Autodesk Fusion 360 part; units mm, degrees
(part 2 of 2)
  spline S185 degree 3 poles (48.0194, -47.8906) (48.2316, -47.8906) (48.3986, -47.7898) (48.5208, -47.5882) knots 0 0 0 0 1 1 1 1
  spline S186 degree 3 poles (48.5208, -47.5882) (48.6431, -47.3867) (48.704, -47.1092) (48.704, -46.7557) knots 0 0 0 0 1 1 1 1
  spline S187 degree 3 poles (48.704, -46.7557) (48.704, -46.4046) (48.6431, -46.1283) (48.5208, -45.9268) knots 0 0 0 0 1 1 1 1
  spline S188 degree 3 poles (48.5208, -45.9268) (48.3986, -45.7252) (48.2316, -45.6244) (48.0194, -45.6244) knots 0 0 0 0 1 1 1 1
  line L174 (46.6928, -45.3714) -> (46.6928, -45.6523)
  line L175 (46.6928, -45.6523) -> (45.7067, -46.5528)
  spline S189 degree 3 poles (45.7067, -46.5528) (45.5889, -46.6608) (45.493, -46.7557) (45.4192, -46.8375) knots 0 0 0 0 1 1 1 1
  spline S190 degree 3 poles (45.4192, -46.8375) (45.3454, -46.9194) (45.2911, -46.9995) (45.2564, -47.0775) knots 0 0 0 0 1 1 1 1
  spline S191 degree 3 poles (45.2564, -47.0775) (45.2216, -47.1557) (45.2043, -47.2419) (45.2043, -47.3362) knots 0 0 0 0 1 1 1 1
  spline S192 degree 3 poles (45.2043, -47.3362) (45.2043, -47.5074) (45.2548, -47.6426) (45.356, -47.7418) knots 0 0 0 0 1 1 1 1
  spline S193 degree 3 poles (45.356, -47.7418) (45.457, -47.841) (45.5957, -47.8906) (45.7718, -47.8906) knots 0 0 0 0 1 1 1 1
  spline S194 degree 3 poles (45.7718, -47.8906) (45.9616, -47.8906) (46.1085, -47.8327) (46.2128, -47.7167) knots 0 0 0 0 1 1 1 1
  spline S195 degree 3 poles (46.2128, -47.7167) (46.317, -47.6007) (46.369, -47.4441) (46.369, -47.2469) knots 0 0 0 0 1 1 1 1
  line L176 (46.369, -47.2469) -> (46.6816, -47.2469)
  spline S196 degree 3 poles (46.6816, -47.2469) (46.6816, -47.4317) (46.6441, -47.5948) (46.5691, -47.7362) knots 0 0 0 0 1 1 1 1
  spline S197 degree 3 poles (46.5691, -47.7362) (46.494, -47.8777) (46.3883, -47.9883) (46.2518, -48.0683) knots 0 0 0 0 1 1 1 1
  spline S198 degree 3 poles (46.2518, -48.0683) (46.1154, -48.1484) (45.956, -48.1883) (45.7737, -48.1883) knots 0 0 0 0 1 1 1 1
  spline S199 degree 3 poles (45.7737, -48.1883) (45.5999, -48.1883) (45.4468, -48.1527) (45.3141, -48.0814) knots 0 0 0 0 1 1 1 1
  spline S200 degree 3 poles (45.3141, -48.0814) (45.1814, -48.0101) (45.0772, -47.9114) (45.0015, -47.7855) knots 0 0 0 0 1 1 1 1
  spline S201 degree 3 poles (45.0015, -47.7855) (44.9259, -47.6596) (44.888, -47.5142) (44.888, -47.3492) knots 0 0 0 0 1 1 1 1
  spline S202 degree 3 poles (44.888, -47.3492) (44.888, -47.1706) (44.9373, -47.0062) (45.036, -46.8561) knots 0 0 0 0 1 1 1 1
  spline S203 degree 3 poles (45.036, -46.8561) (45.1345, -46.7061) (45.2855, -46.5385) (45.489, -46.3537) knots 0 0 0 0 1 1 1 1
  line L177 (45.489, -46.3537) -> (46.2388, -45.6728)
  line L178 (46.2388, -45.6728) -> (46.2388, -45.669)
  line L179 (46.2388, -45.669) -> (44.8712, -45.669)
  line L180 (44.8712, -45.669) -> (44.8712, -45.3714)
  line L181 (44.8712, -45.3714) -> (46.6928, -45.3714)
  spline S204 degree 3 poles (43.6098, -45.3342) (43.7872, -45.3342) (43.9465, -45.371) (44.0879, -45.4448) knots 0 0 0 0 1 1 1 1
  spline S205 degree 3 poles (44.0879, -45.4448) (44.2294, -45.5187) (44.3422, -45.6189) (44.4265, -45.7454) knots 0 0 0 0 1 1 1 1
  spline S206 degree 3 poles (44.4265, -45.7454) (44.5109, -45.8719) (44.5568, -46.0151) (44.5643, -46.1752) knots 0 0 0 0 1 1 1 1
  line L182 (44.5643, -46.1752) -> (44.2294, -46.1752)
  spline S207 degree 3 poles (44.2294, -46.1752) (44.2144, -46.0176) (44.1497, -45.8877) (44.0349, -45.7853) knots 0 0 0 0 1 1 1 1
  spline S208 degree 3 poles (44.0349, -45.7853) (43.9202, -45.683) (43.7785, -45.6319) (43.6098, -45.6319) knots 0 0 0 0 1 1 1 1
  spline S209 degree 3 poles (43.6098, -45.6319) (43.4895, -45.6319) (43.3844, -45.6598) (43.2944, -45.7155) knots 0 0 0 0 1 1 1 1
  spline S210 degree 3 poles (43.2944, -45.7155) (43.2045, -45.7714) (43.134, -45.8481) (43.0832, -45.9453) knots 0 0 0 0 1 1 1 1
  spline S211 degree 3 poles (43.0832, -45.9453) (43.0323, -46.0427) (43.0069, -46.1541) (43.0069, -46.2793) knots 0 0 0 0 1 1 1 1
  spline S212 degree 3 poles (43.0069, -46.2793) (43.0069, -46.4046) (43.0312, -46.5157) (43.0795, -46.6124) knots 0 0 0 0 1 1 1 1
  spline S213 degree 3 poles (43.0795, -46.6124) (43.1279, -46.7092) (43.1955, -46.7851) (43.2823, -46.8403) knots 0 0 0 0 1 1 1 1
  spline S214 degree 3 poles (43.2823, -46.8403) (43.3691, -46.8955) (43.4703, -46.9231) (43.5856, -46.9231) knots 0 0 0 0 1 1 1 1
  spline S215 degree 3 poles (43.5856, -46.9231) (43.7382, -46.9231) (43.869, -46.8924) (43.9782, -46.8311) knots 0 0 0 0 1 1 1 1
  spline S216 degree 3 poles (43.9782, -46.8311) (44.0873, -46.7696) (44.1637, -46.68) (44.207, -46.5622) knots 0 0 0 0 1 1 1 1
  line L183 (44.207, -46.5622) -> (44.5289, -46.5622)
  line L184 (44.5289, -46.5622) -> (44.4359, -48.1436)
  line L185 (44.4359, -48.1436) -> (42.8357, -48.1436)
  line L186 (42.8357, -48.1436) -> (42.8357, -47.846)
  line L187 (42.8357, -47.846) -> (44.1326, -47.846)
  line L188 (44.1326, -47.846) -> (44.1996, -46.9473)
  line L189 (44.1996, -46.9473) -> (44.1959, -46.9473)
  spline S217 degree 3 poles (44.1959, -46.9473) (44.0234, -47.1322) (43.8064, -47.2245) (43.5447, -47.2245) knots 0 0 0 0 1 1 1 1
  spline S218 degree 3 poles (43.5447, -47.2245) (43.3747, -47.2245) (43.225, -47.1843) (43.0953, -47.1036) knots 0 0 0 0 1 1 1 1
  spline S219 degree 3 poles (43.0953, -47.1036) (42.9657, -47.023) (42.8646, -46.9119) (42.792, -46.7705) knots 0 0 0 0 1 1 1 1
  spline S220 degree 3 poles (42.792, -46.7705) (42.7195, -46.6292) (42.6832, -46.4666) (42.6832, -46.2831) knots 0 0 0 0 1 1 1 1
  spline S221 degree 3 poles (42.6832, -46.2831) (42.6832, -46.097) (42.722, -45.9327) (42.7995, -45.7901) knots 0 0 0 0 1 1 1 1
  spline S222 degree 3 poles (42.7995, -45.7901) (42.8771, -45.6474) (42.9852, -45.5358) (43.1242, -45.4551) knots 0 0 0 0 1 1 1 1
  spline S223 degree 3 poles (43.1242, -45.4551) (43.2631, -45.3745) (43.4249, -45.3342) (43.6098, -45.3342) knots 0 0 0 0 1 1 1 1
  spline S224 degree 3 poles (51.1411, -40.5335) (50.8501, -40.5335) (50.6138, -40.2973) (50.6138, -40.0063) knots 0 0 0 0 1 1 1 1
  spline S225 degree 3 poles (50.6138, -40.0063) (50.6138, -39.7153) (50.8501, -39.4791) (51.1411, -39.4791) knots 0 0 0 0 1 1 1 1
  spline S226 degree 3 poles (51.1411, -39.4791) (51.432, -39.4791) (51.6682, -39.7153) (51.6682, -40.0063) knots 0 0 0 0 1 1 1 1
  spline S227 degree 3 poles (51.6682, -40.0063) (51.6682, -40.2973) (51.432, -40.5335) (51.1411, -40.5335) knots 0 0 0 0 1 1 1 1
  spline S228 degree 3 poles (47.5826, -40.6806) (47.2917, -40.6806) (47.0555, -40.4445) (47.0555, -40.1535) knots 0 0 0 0 1 1 1 1
  spline S229 degree 3 poles (47.0555, -40.1535) (47.0555, -39.8626) (47.2917, -39.6263) (47.5826, -39.6263) knots 0 0 0 0 1 1 1 1
  spline S230 degree 3 poles (47.5826, -39.6263) (47.8736, -39.6263) (48.1099, -39.8626) (48.1099, -40.1535) knots 0 0 0 0 1 1 1 1
  spline S231 degree 3 poles (48.1099, -40.1535) (48.1099, -40.4445) (47.8736, -40.6806) (47.5826, -40.6806) knots 0 0 0 0 1 1 1 1
  line L190 (49.9559, -38.0936) -> (50.1177, -38.4567)
  spline S232 degree 3 poles (50.1177, -38.4567) (49.9131, -38.5478) (49.7753, -38.6576) (49.6998, -38.7918) knots 0 0 0 0 1 1 1 1
  spline S233 degree 3 poles (49.6998, -38.7918) (49.6284, -38.9186) (49.6164, -39.0644) (49.6435, -39.2241) knots 0 0 0 0 1 1 1 1
  line L191 (49.6435, -39.2241) -> (49.2597, -39.3221)
  spline S234 degree 3 poles (49.2597, -39.3221) (49.1298, -38.9462) (48.8649, -38.6724) (48.456, -38.506) knots 0 0 0 0 1 1 1 1
  line L192 (48.456, -38.506) -> (48.6058, -38.1377)
  spline S235 degree 3 poles (48.6058, -38.1377) (48.9079, -38.2607) (49.1474, -38.4307) (49.3283, -38.6447) knots 0 0 0 0 1 1 1 1
  spline S236 degree 3 poles (49.3283, -38.6447) (49.3361, -38.6286) (49.3445, -38.6126) (49.3534, -38.5968) knots 0 0 0 0 1 1 1 1
  spline S237 degree 3 poles (49.3534, -38.5968) (49.4641, -38.4002) (49.6561, -38.2272) (49.9559, -38.0936) knots 0 0 0 0 1 1 1 1
extrude "Extrude5" cut sketch "Sketch1 (2)" against normal blind 0.2 contours L8 L9 L10 S0 L11 L12 S1 L13 L14 S2 L15 L16 L17 S3 L18 L19 L20 S4 L21 L22 L23 S5 L24 L25 L26 S6 L27 L28 L29 S7 L30 L31 L32 L33 S8 L34 L35 L36 L37 S9 L38 L39 L40 S10 L41 L42 L43 S11 L44 L45 L46 S12 L47 L48 L49 S13 | S14 S15 S16 L50 S17 S18 S19 S20 S21 S22 L51 S23 S24 S25 S26 S27 S28 S29 S30 L52 S31 S32 S33 S34 S35 S36 S37 L53 S38 S39 S40 S41 S42 | L54 L55 L56 L57 | L58 L59 L60 L61 L62 L63 | L64 L65 L66 L67 L68 L69 L70 L71 | S47 S48 S49 L75 S50 S51 S52 S53 S54 S55 L76 S56 S57 S58 S59 S60 S61 S62 S63 L77 S64 S65 S66 S67 S68 S69 S70 L78 S71 S72 S73 S74 S75 | L79 L80 L81 L82 | L83 L84 L85 L86 S76 S77 L87 L88 L89 L90 L91 L92 L93 L94 L95 | L96 L97 L98 L99 L100 L101 L102 L103 L104 L105 L106 L107 | L108 L109 L110 L111 S78 S79 S80 S81 L112 L113 L114 L115 L116 | L117 L118 S82 S83 S84 S85 S86 S87 L119 L120 L121 | L125 L126 L127 L128 L129 L130 L131 L132 | L136 L137 L138 S96 S97 S98 S99 S100 | L142 L143 L144 L146 L147 L148 L149 | L150 L151 S103 S104 S105 S106 S107 S108 S109 L152 S110 S111 S112 S113 S114 S115 S116 S117 L153 L154 L155 L156 L157 | S118 S119 S120 S121 S122 S123 S124 S125 | S126 S127 S128 L158 S129 S130 S131 S132 S133 S134 S135 S136 S137 S138 L159 L160 L161 L162 L163 L164 L165 S139 S140 S141 S142 S143 S144 S145 | S146 S147 S148 S149 S150 S151 S152 S153 | L166 L167 S154 S155 S156 S157 S158 S159 S160 L168 S161 S162 S163 S164 S165 S166 S167 S168 L169 L170 L171 L172 L173 | S169 S170 S171 S172 S173 S174 S175 S176 S177 S178 S179 S180 | L174 L175 S189 S190 S191 S192 S193 S194 S195 L176 S196 S197 S198 S199 S200 S201 S202 S203 L177 L178 L179 L180 L181 | S204 S205 S206 L182 S207 S208 S209 S210 S211 S212 S213 S214 S215 S216 L183 L184 L185 L186 L187 L188 L189 S217 S218 S219 S220 S221 S222 S223 | S224 S225 S226 S227 | S228 S229 S230 S231 | L190 S232 S233 L191 S234 L192 S235 S236 S237 in component "Hackpad Case"
component "Hackpad Case" placed x (1, 0, 0) y (0, 1, 0) z (0, 0, 1) at (0, 0, 0)
equation "d46 = 3 mm + 15 mm"
